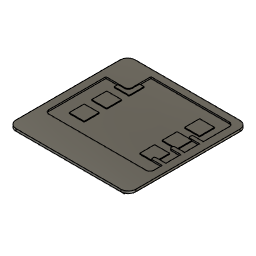
Wall-E-TOP v5 (Autodesk Fusion 360 design; units mm, degrees)
Autodesk Fusion 360 part; units mm, degrees
sketch "Sketch1" plane through (0, 0, 0) normal (0, 0, 1) x (1, 0, 0)
  line L0 (0, 0) -> (139.963, 0)
  line L1 (139.963, 0) -> (139.963, 154)
  line L2 (139.963, 154) -> (0, 154)
  line L3 (0, 154) -> (0, 0)
  dimension "d1" = 139.963
  dimension "d2" = 154
  constraint horizontal L0
  constraint vertical L1
  constraint horizontal L2
  constraint vertical L3
  constraint coincident L0.start L3.end
  measures "d1" distance of L0.start L0.end
  measures "d2" distance of L0.start L2.end
extrude "Extrude1" add sketch "Sketch1" along normal blind 5
sketch "Sketch4" plane through (0, 0, 5) normal (0, 0, 1) x (-1, 0, 0)
  line L0 (0, -154) -> (0, 0)
  line L1 (0, 0) -> (-139.963, 0)
  line L2 (-139.963, 0) -> (-139.963, -154)
  line L3 (-139.963, -154) -> (0, -154)
  line L4 (-139.963, 0) -> (0, -154)
  line L5 (0, 0) -> (-139.963, -154)
  line L6 (10.0185, 0) -> (-149.9815, 0)
  line L7 (-149.9815, 0) -> (-149.9815, -154)
  line L8 (-149.9815, -154) -> (10.0185, -154)
  line L9 (10.0185, -154) -> (10.0185, 0)
  line L10 (10.0185, 0) -> (-149.9815, -154) construction
  line L11 (-149.9815, 0) -> (10.0185, -154) construction
  line L12 (-149.9815, 0) -> (0, 0)
  line L13 (0, 0) -> (0, 5)
  line L14 (0, 5) -> (-149.9815, 5)
  line L15 (-149.9815, 5) -> (-149.9815, 0)
  line L16 (10.0185, 0) -> (0, 0)
  line L17 (0, 0) -> (0, 5)
  line L18 (0, 5) -> (10.0185, 5)
  line L19 (10.0185, 5) -> (10.0185, 0)
  point P0 (-69.9815, -77)
  dimension "d18" = 160
  constraint coincident L1.end L2.start
  constraint coincident L0.start L3.end
  constraint coincident L0.end L1.start
  constraint coincident L2.end L3.start
  constraint horizontal L6
  constraint perpendicular L6 L7
  constraint parallel L6 L8
  constraint parallel L7 L9
  constraint coincident L10 P0
  constraint coincident L11 P0
  constraint midpoint L5 P0
  constraint horizontal L12
  constraint vertical L13
  constraint horizontal L14
  constraint vertical L15
  constraint horizontal L16
  constraint vertical L17
  constraint horizontal L18
  constraint vertical L19
  measures "d18" distance of L7.end L8.end
extrude "Extrude3" add sketch "Sketch4" along normal blind 3
sketch "Sketch5" plane through (0, 0, 8) normal (0, 0, 1) x (-1, 0, 0)
  line L0 (10.0185, 5) -> (-149.9815, 5)
  line L1 (-149.9815, 5) -> (-149.9815, -154)
  line L2 (-149.9815, -154) -> (10.0185, -154)
  line L3 (10.0185, -154) -> (10.0185, 5)
  line L4 (-135, -10) -> (-5, -10)
  line L5 (-5, -10) -> (-5, -140)
  line L6 (-5, -140) -> (-135, -140)
  line L7 (-135, -140) -> (-135, -10)
  constraint horizontal L4
  constraint vertical L5
  constraint horizontal L6
  constraint vertical L7
extrude "Extrude4" cut sketch "Sketch5" against normal blind 2 contours L4 L5 L6 L7
sketch "Sketch6" plane through (0, 0, 8) normal (0, 0, 1) x (-1, 0, 0)
  line L0 (-5, -10) -> (-5, -140)
  line L1 (-5, -140) -> (-135, -140)
  line L2 (-135, -140) -> (-135, -10)
  line L3 (-135, -10) -> (-5, -10)
  line L4 (10.0185, 5) -> (-149.9815, 5)
  line L5 (-149.9815, 5) -> (-149.9815, -154)
  line L6 (-149.9815, -154) -> (10.0185, -154)
  line L7 (10.0185, -154) -> (10.0185, 5)
  line L8 (-135, -10) -> (-5, -10)
  line L9 (-5, -10) -> (-5, -5)
  line L10 (-5, -5) -> (-135, -5)
  line L11 (-135, -5) -> (-135, -10)
  line L12 (-5, -5) -> (0, -5)
  line L13 (0, -5) -> (0, -140)
  line L14 (0, -140) -> (-5, -140)
  line L15 (-5, -140) -> (-5, -5)
  line L16 (-135, -5) -> (-140, -5)
  line L17 (-140, -5) -> (-140, -140)
  line L18 (-140, -140) -> (-135, -140)
  line L19 (-135, -140) -> (-135, -5)
  line L20 (-140, -140) -> (0, -140)
  line L21 (0, -140) -> (0, -145)
  line L22 (0, -145) -> (-140, -145)
  line L23 (-140, -145) -> (-140, -140)
  dimension "d23" = 5
  dimension "d24" = 5
  constraint horizontal L8
  constraint vertical L9
  constraint horizontal L10
  constraint vertical L11
  constraint coincident L2.end L3.start
  constraint horizontal L12
  constraint vertical L13
  constraint horizontal L14
  constraint vertical L15
  constraint horizontal L16
  constraint vertical L17
  constraint horizontal L18
  constraint vertical L19
  constraint horizontal L20
  constraint vertical L21
  constraint horizontal L22
  constraint vertical L23
  measures "d23" distance of L2.end L10.end
  measures "d24" distance of L17.end L22.end
extrude "Extrude5" cut sketch "Sketch6" against normal blind 2 contours L0 L9 L12 L13 L14 L15 L20 | L3 L8 L9 L10 L11 L15 L19 | L1 L14 L18 L20 L21 L22 L23 | L2 L11 L16 L17 L18 L19 L20
sketch "Sketch7" plane through (0, 0, 6) normal (0, 0, 1) x (-1, 0, 0)
  line L0 (0, -5) -> (-140, -5)
  line L1 (-140, -5) -> (-140, -145)
  line L2 (-140, -145) -> (0, -145)
  line L3 (0, -145) -> (0, -5)
  line L4 (-140, -5) -> (0, -5)
  line L5 (0, -5) -> (0, -33.7221)
  line L6 (0, -33.7221) -> (-140, -33.7221)
  line L7 (-140, -33.7221) -> (-140, -5)
  constraint horizontal L4
  constraint vertical L5
  constraint horizontal L6
  constraint vertical L7
  constraint coincident L3 L5.end
  constraint coincident L0.end L1.start
extrude "Extrude6" add sketch "Sketch7" along normal blind 2 contours L0 L1 L3 L4 L5 L6 L7
sketch "Sketch8" plane through (0, 0, 6) normal (0, 0, 1) x (-1, 0, 0)
  line L0 (0, -33.7221) -> (-140, -33.7221)
  line L1 (-140, -33.7221) -> (-140, -145)
  line L2 (-140, -145) -> (0, -145)
  line L3 (0, -145) -> (0, -33.7221)
  line L4 (0, -145) -> (-30, -145)
  line L5 (-30, -145) -> (-30, -115)
  line L6 (-30, -115) -> (0, -115)
  line L7 (0, -115) -> (0, -145)
  constraint horizontal L4
  constraint vertical L5
  constraint horizontal L6
  constraint vertical L7
  constraint coincident L2.end L3.start
extrude "Extrude7" add sketch "Sketch8" along normal blind 2 contours L2 L3 L4 L5 L6 L7
sketch "Sketch9" plane through (0, 0, 6) normal (0, 0, 1) x (-1, 0, 0)
  line L0 (-30, -145) -> (-30, -115)
  line L1 (-30, -115) -> (0, -115)
  line L2 (0, -115) -> (0, -33.7221)
  line L3 (0, -33.7221) -> (-140, -33.7221)
  line L4 (-140, -33.7221) -> (-140, -145)
  line L5 (-140, -145) -> (-30, -145)
  line L6 (-140, -100) -> (-125, -100)
  line L7 (-125, -100) -> (-125, -105)
  line L8 (-125, -105) -> (-140, -105)
  line L9 (-140, -105) -> (-140, -100)
  line L10 (-140, -75) -> (-125, -75)
  line L11 (-125, -75) -> (-125, -80)
  line L12 (-125, -80) -> (-140, -80)
  line L13 (-140, -80) -> (-140, -75)
  line L14 (-140, -50) -> (-125, -50)
  line L15 (-125, -50) -> (-125, -55)
  line L16 (-125, -55) -> (-140, -55)
  line L17 (-140, -55) -> (-140, -50)
  constraint horizontal L6
  constraint vertical L7
  constraint horizontal L8
  constraint vertical L9
  constraint coincident L4 L6.start
  constraint horizontal L10
  constraint vertical L11
  constraint horizontal L12
  constraint vertical L13
  constraint coincident L4 L10.start
  constraint horizontal L14
  constraint vertical L15
  constraint horizontal L16
  constraint vertical L17
  constraint coincident L4 L14.start
extrude "Extrude8" add sketch "Sketch9" along normal blind 2 contours L4 L6 L7 L8 L9 | L4 L10 L11 L12 L13 | L4 L14 L15 L16 L17
fillet "Fillet3" radius 5 4 edges at (0, 33.7221, 7) (140, 33.7221, 7) (140, 145, 7) (30, 115, 7)
fillet "Fillet4" radius 2 6 edges at (125, 55, 7) (125, 80, 7) (125, 105, 7) (125, 100, 7) (125, 75, 7) (125, 50, 7)
sketch "Sketch10" plane through (0, 0, 6) normal (0, 0, 1) x (-1, 0, 0)
  arc A0 (-140, -140) -> (-135, -145) centre (-135, -140) ccw
  line L0 (-135, -145) -> (-30, -145)
  line L1 (-30, -145) -> (-30, -120)
  arc A1 (-25, -115) -> (-30, -120) centre (-25, -120) ccw
  line L2 (-25, -115) -> (0, -115)
  line L3 (0, -115) -> (0, -38.7221)
  arc A2 (0, -38.7221) -> (-5, -33.7221) centre (-5, -38.7221) ccw
  line L4 (-5, -33.7221) -> (-135, -33.7221)
  arc A3 (-135, -33.7221) -> (-140, -38.7221) centre (-135, -38.7221) ccw
  line L5 (-140, -38.7221) -> (-140, -50)
  line L6 (-140, -50) -> (-127, -50)
  arc A4 (-125, -52) -> (-127, -50) centre (-127, -52) ccw
  line L7 (-125, -52) -> (-125, -53)
  arc A5 (-127, -55) -> (-125, -53) centre (-127, -53) ccw
  line L8 (-127, -55) -> (-140, -55)
  line L9 (-140, -55) -> (-140, -75)
  line L10 (-140, -75) -> (-127, -75)
  arc A6 (-125, -77) -> (-127, -75) centre (-127, -77) ccw
  line L11 (-125, -77) -> (-125, -78)
  arc A7 (-127, -80) -> (-125, -78) centre (-127, -78) ccw
  line L12 (-127, -80) -> (-140, -80)
  line L13 (-140, -80) -> (-140, -100)
  line L14 (-140, -100) -> (-127, -100)
  arc A8 (-125, -102) -> (-127, -100) centre (-127, -102) ccw
  line L15 (-125, -102) -> (-125, -103)
  arc A9 (-127, -105) -> (-125, -103) centre (-127, -103) ccw
  line L16 (-127, -105) -> (-140, -105)
  line L17 (-140, -105) -> (-140, -140)
  line L18 (-130, -130) -> (-110, -130)
  line L19 (-110, -130) -> (-110, -110)
  line L20 (-110, -110) -> (-130, -110)
  line L21 (-130, -110) -> (-130, -130)
  line L22 (-40, -50) -> (-20, -50)
  line L23 (-20, -50) -> (-20, -70)
  line L24 (-20, -70) -> (-40, -70)
  line L25 (-40, -70) -> (-40, -50)
  line L26 (-40, -80) -> (-20, -80)
  line L27 (-20, -80) -> (-20, -100)
  line L28 (-20, -100) -> (-40, -100)
  line L29 (-40, -100) -> (-40, -80)
  line L30 (-40, -110) -> (-20, -110)
  line L31 (-20, -110) -> (-20, -130)
  line L32 (-20, -130) -> (-40, -130)
  line L33 (-40, -130) -> (-40, -110)
  line L34 (-130, -100) -> (-110, -100)
  line L35 (-110, -100) -> (-110, -80)
  line L36 (-110, -80) -> (-130, -80)
  line L37 (-130, -80) -> (-130, -100)
  line L38 (-130, -70) -> (-110, -70)
  line L39 (-110, -70) -> (-110, -50)
  line L40 (-110, -50) -> (-130, -50)
  line L41 (-130, -50) -> (-130, -70)
  constraint horizontal L18
  constraint vertical L19
  constraint horizontal L20
  constraint vertical L21
  constraint horizontal L22
  constraint vertical L23
  constraint horizontal L24
  constraint vertical L25
  constraint horizontal L26
  constraint vertical L27
  constraint horizontal L28
  constraint vertical L29
  constraint horizontal L30
  constraint vertical L31
  constraint horizontal L32
  constraint vertical L33
  constraint horizontal L34
  constraint vertical L35
  constraint horizontal L36
  constraint vertical L37
  constraint coincident L14 L34.start
  constraint horizontal L38
  constraint vertical L39
  constraint horizontal L40
  constraint vertical L41
extrude "Extrude9" add sketch "Sketch10" along normal blind 1 contours L1 A1 L2 L30 L31 L32 L33 | L12 L14 L34 L35 L36 L37 | A4 L7 A5 L8 L38 L39 L40 L41 | L18 L19 L20 L21 | L22 L23 L24 L25 | L26 L27 L28 L29
fillet "Fillet5" radius 10 4 edges at (149.9815, 154, 6.5) (-10.0185, 154, 6.5) (149.9815, -5, 6.5) (-10.0185, -5, 6.5)
move_face "MoveFace1" by (-15, 0, 0) 1 faces at (33.3333, 56.6667, 7)
move_face "MoveFace2" by (-15, 0, 0) 1 faces at (33.3333, 56.6667, 7)
extrude "Extrude10" add 3 faces at (20, 111.6667, 6.3333) (20, 86.6667, 6.3333) (20, 56.6667, 6.3333) along direction (-1, 0, 0) blind 4
extrude "Extrude11" cut 3 faces at (40, 123.3333, 6.3333) (40, 93.3333, 6.3333) (40, 63.3333, 6.3333) along direction (-1, 0, 0) blind 4
